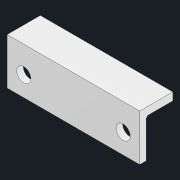
# Autodesk Inventor part: base38
Saved by Autodesk Inventor 2021 (Build 250183000, 183)
## iProperties
Created: 2021-08-07
Part Number: base38
Material: ABS プラスチック
Document SubType Name: Modeling
Designer: yuta0
Density: 1.06 g/cm^3
Appearance: 滑らか - 白
Mass: 1.92173 g
Surface Area: 20.095 cm^2
Volume: 1.81295 cm^3
在庫数: 0.0
購入先: 印刷
Author: yuta0
Autodesk Inventor part; units mm, degrees
ref_plane "YZ Plane" through (0, 0, 0) normal (1, 0, 0) x (0, 1, 0)
ref_plane "XZ Plane" through (0, 0, 0) normal (0, 1, 0) x (-1, 0, 0)
ref_plane "XY Plane" through (0, 0, 0) normal (0, 0, 1) x (1, 0, 0)
sketch "スケッチ1" plane through (0, 0, 0) normal (0, 0, 1) x (1, 0, 0)
  line L0 (-20, -6) -> (20, -6)
  line L1 (20, -6) -> (20, 8)
  line L2 (20, 8) -> (-20, 8)
  line L3 (-20, 8) -> (-20, -6)
  point P0 (0, 0)
  dimension "d1" = 40
  dimension "d21" = 8
  dimension "d22" = 6
  dimension "d23" = 20
  constraints: 8 end point, 2 parallel, 1 horizontal, 1 perpendicular
  measures "d1" distance of L1.end L2.end
  measures "d21" distance from line of L2 point (0, 0)
  measures "d22" distance from line of L0 point (0, 0)
  measures "d23" distance from line of L3 point (0, 0)
extrude "押し出し1" add sketch "スケッチ1" along normal blind 2
sketch "スケッチ2" plane through (0, 0, 2) normal (0, 0, 1) x (1, 0, 0)
  line L0 (-20, -6) -> (20, -6) projected
  point P0 (0, 0)
  point P1 (-15, 0)
  point P2 (15, 0)
  dimension "d4" = 6
  dimension "d5" = 6
  dimension "d24" = 15
  dimension "d25" = 15
  measures "d4" distance from line of L0 point (-15, 0)
  measures "d5" distance from line of L0 point (15, 0)
  measures "d24" distance of point (0, 0) point (-15, 0)
  measures "d25" distance of point (15, 0) point (0, 0)
hole "穴1" at (-15, 0, 2) at (15, 0, 2) direction (0, 0, -1) diameter 4.3 end through all clearance for "Flat Head Machine Screw" size "M4" standard "Ansi Metric M Profile"
sketch "スケッチ3" plane through (0, 0, 0) normal (0, 0, -1) x (-1, 0, 0)
  circle A0 centre (15, 0) radius 2.15 projected
  circle A1 centre (-15, 0) radius 2.15 projected
  line L0 (-20, -6) -> (-20, 8) projected
  line L1 (20, -6) -> (-20, -6) projected
  line L2 (20, 8) -> (20, -6) projected
  line L3 (-20, 8) -> (20, 8) projected
  line L4 (-20, 8) -> (20, 8)
  line L5 (20, 8) -> (20, 5.653)
  line L6 (20, 5.653) -> (-20, 5.653)
  line L7 (-20, 5.653) -> (-20, 8)
  point P0 (0, 0)
  point P1 (-20, 5.653)
  dimension "d15" = 2.347
  constraints: 8 end point, 2 parallel, 1 horizontal, 1 perpendicular, 1 point on line
  measures "d15" distance between parallel lines of L3 L6
extrude "押し出し2" add sketch "スケッチ3" along normal blind 8 contours L0 L3 L2 L6
chamfer "面取り2" distance 0.5 angle 45 1 edges at (0, 5.653, 0)
